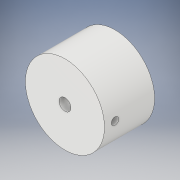
# Autodesk Inventor part: AA009
Saved by Autodesk Inventor 2017 SP1 (Build 210196100, 196)
## iProperties
Created: 2017-07-19
Part Number: AA009
Material: ABS Plastic
Document SubType Name: Modeling
Designer: Zach
Density: 1.06 g/cm^3
Appearance: CR White
Author: Zach
Autodesk Inventor part; units mm, degrees
ref_plane "YZ Plane" through (0, 0, 0) normal (1, 0, 0) x (0, 1, 0)
ref_plane "XZ Plane" through (0, 0, 0) normal (0, 1, 0) x (-1, 0, 0)
ref_plane "XY Plane" through (0, 0, 0) normal (0, 0, 1) x (1, 0, 0)
sketch "Sketch1" plane through (0, 0, 0) normal (0, 0, 1) x (1, 0, 0)
  circle A0 centre (0, 0) radius 15
  dimension "d0" = 30
  constraints: 1 centre point, 1 coincident
  measures "d0" diameter of A0
extrude "Extrusion1" add sketch "Sketch1" along normal blind 14
sketch "Sketch2" plane through (0, 0, 14) normal (0, 0, 1) x (1, 0, 0)
  circle A0 centre (0, 0) radius 2.25
  dimension "d3" = 4.5
  constraints: 1 centre point, 1 coincident
  measures "d3" diameter of A0
extrude "Extrusion2" cut sketch "Sketch2" against normal blind 19
sketch "Sketch3" plane through (0, 0, 0) normal (0, 0, -1) x (-1, 0, 0)
  circle A0 centre (0, 0) radius 15 projected
extrude "Extrusion3" add sketch "Sketch3" along normal blind 5
sketch "Sketch6" plane through (0, 0, -5) normal (0, 0, -1) x (-1, 0, 0)
  line L0 (0, -8) -> (-6.9282, -4)
  line L1 (-6.9282, -4) -> (-6.9282, 4)
  line L2 (-6.9282, 4) -> (0, 8)
  line L3 (0, 8) -> (6.9282, 4)
  line L4 (6.9282, 4) -> (6.9282, -4)
  line L5 (6.9282, -4) -> (0, -8)
  point P0 (0, 0)
  point P1 (0, 0)
  dimension "d15" = 16
  constraints: 12 end point, 1 coincident, 13 other
  measures "d15" distance of L0.start L2.end
extrude "Extrusion6" cut sketch "Sketch6" against normal blind 5
sketch "Sketch7" plane through (0, 0, 0) normal (1, 0, 0) x (0, 1, 0)
  circle A0 centre (0, 10) radius 1.4
  line L0 (15, 14) -> (-15, 14) projected
  point P0 (0, 0)
  dimension "d18" = 2.8
  dimension "d22" = 4
  constraints: 1 centre point, 1 vertical alignment
  measures "d18" diameter of A0
  measures "d22" distance from line of L0 A0.centre
extrude "Extrusion7" cut sketch "Sketch7" along normal through all
body "Solid1"
